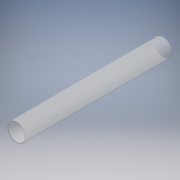
# Autodesk Inventor part: Tube Lanceur
Saved by Autodesk Inventor 2016 SP1 (Build 200210100, 210)
## iProperties
Created: 2017-04-25
Part Number: Tube Lanceur
Material: Plastique PMMA
Document SubType Name: Modeling
Designer: dimercur
Density: 1.188 g/cm^3
Appearance: Transparent - Clair
Author: dimercur
Autodesk Inventor part; units mm, degrees
ref_plane "YZ Plane" through (0, 0, 0) normal (1, 0, 0) x (0, 1, 0)
ref_plane "XZ Plane" through (0, 0, 0) normal (0, 1, 0) x (-1, 0, 0)
ref_plane "XY Plane" through (0, 0, 0) normal (0, 0, 1) x (1, 0, 0)
sketch "Esquisse1" plane through (0, 0, 0) normal (0, 1, 0) x (-1, 0, 0)
  circle A0 centre (0, 0) radius 25
  circle A1 centre (0, 0) radius 22.5
  dimension "d0" = 50
  dimension "d1" = 2.5
  constraints: 2 centre point, 2 coincident
  measures "d0" diameter of A0
  measures "d1" radial gap between concentric circles of A1 A0
extrude "Extrusion1" add sketch "Esquisse1" along normal blind 400
